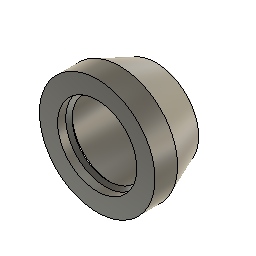
gromet (Autodesk Fusion 360 design; units mm, degrees)
Autodesk Fusion 360 part; units mm, degrees
sketch "Sketch1" plane through (0, 0, 0) normal (0, 0, 1) x (1, 0, 0)
  line L0 (4.9, 0) -> (4.9, 1)
  line L1 (4.9, 1) -> (4.5, 1.4)
  line L2 (4.5, 1.4) -> (4.9, 1.8)
  line L3 (4.9, 1.8) -> (4.9, 8.2)
  line L4 (4.9, 8.2) -> (7.15, 2.8)
  line L5 (7.15, 2.8) -> (7.15, 0)
  line L6 (7.15, 0) -> (4.9, 0)
  dimension "d1" = 4.9
  dimension "d3" = 2.25
  dimension "d6" = 2.8
  dimension "d7" = 8.2
  dimension "d8" = 90
  dimension "d10" = 0.8
  dimension "d11" = 1.4
  constraint vertical L0
  constraint parallel L0 L3
  constraint parallel L3 L5
  constraint perpendicular L0 L6
  constraint coincident origin L6
  constraint coincident L3.end L4.start
  constraint collinear L0 L3
  constraint equal L1 L2
  measures "d1" distance of origin L0.start
  measures "d3" distance of L0.start L5.end
  measures "d6" distance of L4.end L5.end
  measures "d7" vertical distance of L0.start L3.end
  measures "d8" angle of L1 L2
  measures "d10" distance of L0.end L2.end
  measures "d11" vertical distance of L0.start L1.end
revolve "Revolve1" add sketch "Sketch1" angle 360 about axis through (0, 1.75, 0) along (0, 1, 0)
fillet "Fillet1" radius 0.2 tangency weight 1.5 1 edges at (-4.5684, 8.2, -1.7719)
equation "d1 = InnerDiameter / 2 - Tolerance"
equation "Tolerance = 0.1 mm"
equation "d3 = ( OuterDiameter - InnerDiameter ) / 2"
equation "InnerDiameter = 10 mm"
equation "OuterDiameter = 14.50 mm"
equation "d7 = 2.6 mm + 5.6 mm"
equation "d11 = ( 2.8 / 2 ) * 1 mm"
